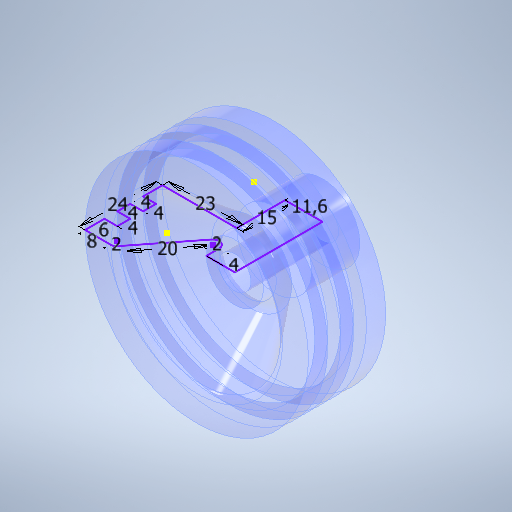
# Autodesk Inventor part: pierścień_uszczelniający
Saved by Autodesk Inventor 2025 (Build 290162000, 162)
## iProperties
Created: 2025-03-16
Part Number: pierścień_uszczelniający
Material: Tworzywo sztuczne PET
Document SubType Name: Modeling
Designer: barte
Density: 1.541 g/cm^3
Appearance: Przezroczysty — niebieski
Author: barte
Autodesk Inventor part; units mm, degrees
ref_plane "YZ Plane" through (0, 0, 0) normal (1, 0, 0) x (0, 1, 0)
ref_plane "XZ Plane" through (0, 0, 0) normal (0, 1, 0) x (-1, 0, 0)
ref_plane "XY Plane" through (0, 0, 0) normal (0, 0, 1) x (1, 0, 0)
sketch "Szkic1" plane through (0, 0, 0) normal (0, 1, 0) x (-1, 0, 0)
  line L0 (5.43, 11.8473) -> (13.43, 11.8473)
  line L1 (13.43, -12.1527) -> (-9.57, -12.1527)
  line L2 (-9.57, -12.1527) -> (-9.57, -27.1527)
  line L3 (-9.57, -27.1527) -> (-21.17, -27.1527)
  arc A0 (5.43, 11.8473) -> (3.5548, 10.5426) centre (5.43, 9.8473) ccw
  line L4 (3.5548, 10.5426) -> (-8.7625, -5.2144)
  arc A1 (-12.3382, -3.9827) -> (-8.7625, -5.2144) centre (-10.3382, -3.9827) ccw
  line L5 (-12.3382, -3.9827) -> (-12.3382, 0.0173)
  line L6 (-21.17, -27.1527) -> (-21.17, 0.0173)
  line L7 (-21.17, 0.0173) -> (-12.3382, 0.0173)
  line L8 (13.43, 11.8473) -> (13.43, 5.8473)
  line L9 (13.43, 5.8473) -> (9.43, 5.8473)
  line L10 (9.43, 5.8473) -> (9.43, 1.8473)
  line L11 (9.43, 1.8473) -> (13.43, 1.8473)
  line L12 (13.43, 1.8473) -> (13.43, -2.1527)
  line L13 (13.43, -2.1527) -> (9.43, -2.1527)
  line L14 (9.43, -2.1527) -> (9.43, -6.1527)
  line L15 (9.43, -6.1527) -> (13.43, -6.1527)
  line L16 (13.43, -6.1527) -> (13.43, -12.1527)
  point P0 (0, 0)
  dimension "d0" = 8
  dimension "d1" = 24
  dimension "d2" = 23
  dimension "d3" = 15
  dimension "d4" = 11.6
  dimension "d5" = 2
  dimension "d6" = 20
  dimension "d7" = 2
  dimension "d8" = 4
  dimension "d13" = 6
  dimension "d15" = 4
  dimension "d16" = 4
  dimension "d17" = 4
  dimension "d18" = 4
  constraints: 34 end point, 5 perpendicular, 4 point on circle, 3 tangent, 2 centre point, 2 point on line, 2 vertical, 1 horizontal
  measures "d0" distance of L0.start L0.end
  measures "d1" distance of L0.end L1.start
  measures "d2" distance of L1.start L1.end
  measures "d3" distance of L1.end L2.end
  measures "d4" distance of L2.end L3.end
  measures "d5" radius of A0
  measures "d6" distance of L4.start L4.end
  measures "d7" radius of A1
  measures "d8" distance of L5.end L5.start
  measures "d13" distance of L0.end L8.end
  measures "d15" distance of L9.end L10.end
  measures "d16" distance of L11.end L12.end
  measures "d17" distance of L12.end L13.end
  measures "d18" distance of L13.end L14.end
revolve "Obrót1" add sketch "Szkic1" angle 360 about axis through (21.17, 0, -27.1527) along (0, 0, 1)
sketch "Szkic2" plane through (21.17, 0, -27.1527) normal (0, 0, -1) x (-1, 0, 0)
  point P0 (21.17, 0)
sketch "Szkic3" plane through (21.17, 0, -27.1527) normal (0, 0, -1) x (-1, 0, 0)
  circle A0 centre (0, 0) radius 5
  point P0 (21.17, 0)
  dimension "d10" = 10
  constraints: 1 centre point
  measures "d10" diameter of A0
sketch "Szkic4" plane through (21.17, 0, -27.1527) normal (0, 0, -1) x (-1, 0, 0)
  point P0 (21.17, 0)
extrude "Wyciągnięcie proste1" cut sketch "Szkic3" against normal blind 39
